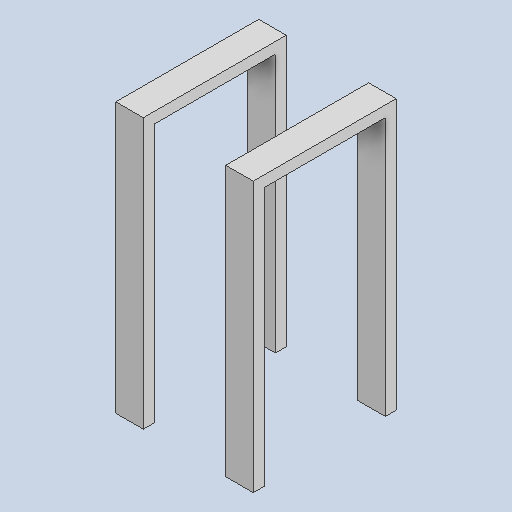
# Autodesk Inventor part: Bridge
Saved by Autodesk Inventor 2022 (Build 260153000, 153)
## iProperties
Created: 2021-11-08
Part Number: Bridge
Material: Generisch
Document SubType Name: Modeling
Designer: lukas
Density: 1 g/cm^3
Appearance: Vorgabe
Author: lukas
Autodesk Inventor part; units mm, degrees
ref_plane "YZ Plane" through (0, 0, 0) normal (1, 0, 0) x (0, 1, 0)
ref_plane "XZ Plane" through (0, 0, 0) normal (0, 1, 0) x (-1, 0, 0)
ref_plane "XY Plane" through (0, 0, 0) normal (0, 0, 1) x (1, 0, 0)
sketch "Skizze1" plane through (0, 0, 0) normal (0, 1, 0) x (-1, 0, 0)
  line L0 (-26.5441, -1.2228) -> (-26.5441, 24.7772) projected
  line L1 (-28.5441, 26.7772) -> (-82.5441, 26.7772) projected
  line L2 (-84.5441, 4.8607) -> (-84.5441, -1.2228) projected
  line L3 (-82.5441, -3.2228) -> (-28.5441, -3.2228) projected
  line L4 (-32.5441, -1.2228) -> (-78.5441, -1.2228) projected
  line L5 (-82.5441, 18.6937) -> (-82.5441, 21.7772) projected
  line L6 (-78.5441, 24.7772) -> (-32.5441, 24.7772) projected
  line L7 (-28.5441, 21.7772) -> (-28.5441, 1.7772) projected
  line L8 (-71.5441, 12.2772) -> (-71.5441, 11.2772) projected
  line L9 (-66.5441, 0.7522) -> (-71.5441, 0.7522)
  line L10 (-71.5441, 0.7522) -> (-71.5441, -1.2228)
  line L11 (-71.5441, -1.2228) -> (-66.5441, -1.2228)
  line L12 (-66.5441, -1.2228) -> (-66.5441, 0.7522)
  line L13 (-66.5441, 22.8022) -> (-71.5441, 22.8022)
  line L14 (-71.5441, 22.8022) -> (-71.5441, 24.7772)
  line L15 (-71.5441, 24.7772) -> (-66.5441, 24.7772)
  line L16 (-66.5441, 24.7772) -> (-66.5441, 22.8022)
  line L17 (-51.5441, 0.7522) -> (-46.5441, 0.7522)
  line L18 (-46.5441, 0.7522) -> (-46.5441, -1.2228)
  line L19 (-46.5441, -1.2228) -> (-51.5441, -1.2228)
  line L20 (-51.5441, -1.2228) -> (-51.5441, 0.7522)
  line L21 (-51.5441, 22.8022) -> (-46.5441, 22.8022)
  line L22 (-46.5441, 22.8022) -> (-46.5441, 24.7772)
  line L23 (-46.5441, 24.7772) -> (-51.5441, 24.7772)
  line L24 (-51.5441, 24.7772) -> (-51.5441, 22.8022)
  arc A0 (-60.2341, 17.4772) -> (-60.4341, 18.349) centre (-62.2341, 17.4772) ccw projected
  arc A1 (-60.4341, 5.2054) -> (-60.2341, 6.0772) centre (-62.2341, 6.0772) ccw projected
  arc A2 (-60.2341, 17.4772) -> (-60.4341, 18.349) centre (-62.2341, 17.4772) ccw projected
  arc A3 (-60.4341, 5.2054) -> (-60.2341, 6.0772) centre (-62.2341, 6.0772) ccw projected
  line L25 (-28.5441, 8.0272) -> (-28.5441, 24.7772) projected
  line L26 (-29.4341, 3.0272) -> (-29.4341, 8.0272) projected
  line L27 (-30.2441, 20.5272) -> (-60.4341, 20.5272) projected
  line L28 (-60.4341, 20.5272) -> (-60.4341, 18.349) projected
  line L29 (-60.4341, 5.2054) -> (-60.4341, 3.0272) projected
  line L30 (-60.4341, 3.0272) -> (-29.4341, 3.0272) projected
  line L31 (-29.4341, 8.0272) -> (-28.5441, 8.0272) projected
  line L32 (-28.5441, 8.0272) -> (-28.5441, 24.7772) projected
  line L33 (-29.4341, 3.0272) -> (-29.4341, 8.0272) projected
  line L34 (-30.2441, 20.5272) -> (-60.4341, 20.5272) projected
  line L35 (-60.4341, 20.5272) -> (-60.4341, 18.349) projected
  line L36 (-60.4341, 5.2054) -> (-60.4341, 3.0272) projected
  line L37 (-60.4341, 3.0272) -> (-29.4341, 3.0272) projected
  line L38 (-29.4341, 8.0272) -> (-28.5441, 8.0272) projected
  line L39 (-30.2441, 24.7772) -> (-30.2441, 20.5272) projected
  line L40 (-30.2441, 24.7772) -> (-30.2441, 20.5272) projected
  line L41 (-28.5441, 24.7772) -> (-30.2441, 24.7772) projected
  line L42 (-28.5441, 24.7772) -> (-30.2441, 24.7772) projected
  line L43 (-82.5441, 4.8607) -> (-84.5441, 4.8607) projected
  line L44 (-84.5441, 24.7772) -> (-84.5441, 18.6937) projected
  line L45 (-84.5441, 18.6937) -> (-82.5441, 18.6937) projected
  line L46 (-82.5441, 1.7772) -> (-82.5441, 4.8607) projected
  arc A4 (-82.5441, 26.7772) -> (-84.5441, 24.7772) centre (-82.5441, 24.7772) ccw projected
  line L47 (-82.5441, 21.7772) -> (-78.5441, 21.7772) projected
  line L48 (-78.5441, 24.7772) -> (-78.5441, 21.7772) projected
  line L49 (-32.5441, 21.7772) -> (-32.5441, 24.7772) projected
  line L50 (-28.5441, 21.7772) -> (-32.5441, 21.7772) projected
  line L51 (-28.5441, 1.7772) -> (-32.5441, 1.7772) projected
  line L52 (-32.5441, -1.2228) -> (-32.5441, 1.7772) projected
  line L53 (-78.5441, 1.7772) -> (-78.5441, -1.2228) projected
  line L54 (-82.5441, 1.7772) -> (-78.5441, 1.7772) projected
  arc A5 (-84.5441, -1.2228) -> (-82.5441, -3.2228) centre (-82.5441, -1.2228) ccw projected
  arc A6 (-28.5441, -3.2228) -> (-26.5441, -1.2228) centre (-28.5441, -1.2228) ccw projected
  arc A7 (-26.5441, 24.7772) -> (-28.5441, 26.7772) centre (-28.5441, 24.7772) ccw projected
  circle A8 centre (-29.5441, -0.7228) radius 1.6 projected
  circle A9 centre (-81.5441, -0.7228) radius 1.6 projected
  circle A10 centre (-29.5441, 24.2772) radius 1.6 projected
  circle A11 centre (-81.5441, 24.2772) radius 1.6 projected
  line L55 (-60.2341, 17.4772) -> (-60.2341, 6.0772) projected
  line L56 (-60.2341, 17.4772) -> (-60.2341, 6.0772) projected
  point P0 (0, 0)
  point P1 (-82.5441, 23.9022)
  point P2 (-16.5441, 23.9022)
  point P3 (-82.5441, -0.3478)
  point P4 (-16.5441, -0.3478)
  point P5 (-46.5441, -1.2228)
  point P6 (-34.1441, -1.2228)
  point P7 (-34.1441, 24.7772)
  point P8 (-82.5441, 21.7022)
  point P9 (-82.5441, 14.9472)
  point P10 (-84.5441, 14.9472)
  point P11 (-84.5441, 8.6072)
  point P12 (-82.5441, 8.6072)
  point P13 (-82.5441, 1.8522)
  point P14 (-62.2341, 17.4772)
  point P15 (-62.2341, 6.0772)
  point P16 (-62.2341, 17.4772)
  point P17 (-62.2341, 6.0772)
  point P18 (-28.4341, -1.2228)
  point P19 (-28.4341, 24.7772)
  point P20 (-62.2341, 17.4772)
  point P21 (-62.2341, 6.0772)
  point P22 (-62.2341, 17.4772)
  point P23 (-62.2341, 6.0772)
  point P24 (-62.2341, 17.4772)
  point P25 (-62.2341, 6.0772)
  point P26 (-62.2341, 17.4772)
  point P27 (-62.2341, 6.0772)
  point P28 (-62.2341, 17.4772)
  point P29 (-62.2341, 6.0772)
  point P30 (-62.2341, 17.4772)
  point P31 (-62.2341, 6.0772)
  point P32 (-62.2341, 17.4772)
  point P33 (-62.2341, 6.0772)
  point P34 (-62.2341, 17.4772)
  point P35 (-62.2341, 6.0772)
  point P36 (-62.2341, 17.4772)
  point P37 (-62.2341, 6.0772)
  point P38 (-62.2341, 17.4772)
  point P39 (-62.2341, 6.0772)
  constraints: 32 end point, 8 parallel, 4 horizontal, 4 perpendicular, 2 point on line, 3 other
extrude "Extrusion1" add sketch "Skizze1" along normal blind 47.0872 contours L10 L9 L12 L4 | L6 L16 L13 L14 | L20 L17 L18 L4 | L6 L22 L21 L24
sketch "Skizze2" plane through (0, 47.0872, 0) normal (0, 1, 0) x (1, 0, 0)
  line L0 (71.5441, 1.2228) -> (66.5441, 1.2228) projected
  line L1 (71.5441, -0.7522) -> (71.5441, 1.2228) projected
  line L2 (66.5441, -24.7772) -> (71.5441, -24.7772)
  line L3 (71.5441, -24.7772) -> (71.5441, 1.2228)
  line L4 (71.5441, 1.2228) -> (66.5441, 1.2228)
  line L5 (66.5441, 1.2228) -> (66.5441, -24.7772)
  line L6 (51.5441, 1.2228) -> (46.5441, 1.2228) projected
  line L7 (51.5441, 1.2228) -> (46.5441, 1.2228)
  line L8 (46.5441, 1.2228) -> (46.5441, -24.7772)
  line L9 (46.5441, -24.7772) -> (51.5441, -24.7772)
  line L10 (51.5441, -24.7772) -> (51.5441, 1.2228)
  line L11 (46.5441, -0.7522) -> (51.5441, -0.7522) projected
  line L12 (51.5441, -0.7522) -> (51.5441, 1.2228) projected
  line L13 (51.5441, 1.2228) -> (46.5441, 1.2228) projected
  line L14 (46.5441, 1.2228) -> (46.5441, -0.7522) projected
  line L15 (71.5441, 1.2228) -> (66.5441, 1.2228) projected
  line L16 (66.5441, 1.2228) -> (66.5441, -0.7522) projected
  line L17 (66.5441, -0.7522) -> (71.5441, -0.7522) projected
  line L18 (71.5441, -0.7522) -> (71.5441, 1.2228) projected
  line L19 (46.5441, -24.7772) -> (51.5441, -24.7772) projected
  line L20 (51.5441, -24.7772) -> (51.5441, -22.8022) projected
  line L21 (51.5441, -22.8022) -> (46.5441, -22.8022) projected
  line L22 (46.5441, -22.8022) -> (46.5441, -24.7772) projected
  line L23 (71.5441, -22.8022) -> (66.5441, -22.8022) projected
  line L24 (66.5441, -22.8022) -> (66.5441, -24.7772) projected
  line L25 (66.5441, -24.7772) -> (71.5441, -24.7772) projected
  line L26 (71.5441, -24.7772) -> (71.5441, -22.8022) projected
  point P0 (0, 0)
  constraints: 16 end point, 4 parallel, 2 horizontal, 2 perpendicular
extrude "Extrusion2" add sketch "Skizze2" along normal blind 2
